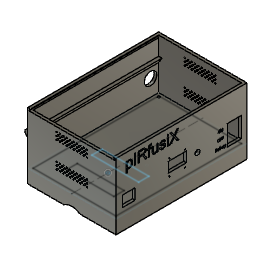
Gateway Enclosure Final Version (Autodesk Fusion 360 design; units mm, degrees)
Autodesk Fusion 360 part; units mm, degrees
(part 1 of 2)
box "BoxPrimitive1" add length 193 width 130 height 77.5 placed x (0, 1, 0) y (-1, 0, 0) z (0, 0, 1) at (80, 0, 0) makes body 1 in component "Box"
shell "Shell1" thickness 4 removed faces 1 at (36.6667, 64.3333, 77.5) on bodies 1 in component "Box"
sketch "Sketch2" plane through (0, 0, 0) normal (0, -1, 0) x (1, 0, 0) in component "Box"
  line L0 (-50, 77.5) -> (-50, 0)
  line L1 (-50, 0) -> (80, 0)
  line L2 (80, 0) -> (80, 77.5)
  line L3 (80, 77.5) -> (-50, 77.5)
  line L4 (76, 77.5) -> (78.2943, 74.2234)
  line L5 (76, 77.5) -> (80, 77.5) construction
  line L6 (15, 77.5) -> (15, 74.2234) construction
  line L7 (15, 74.2234) -> (78.2943, 74.2234)
  line L8 (15, 74.2234) -> (-48.2943, 74.2234)
  line L9 (-46, 77.5) -> (-48.2943, 74.2234)
  point P0 (-46, 77.5)
  point P1 (76, 77.5)
  dimension "d7" = 55
  dimension "d8" = 4
  constraint horizontal L5
  constraint coincident P1 L4.start
  constraint coincident L2.end L3.start
  constraint midpoint L3 L6.start
  constraint perpendicular L3 L6
  constraint horizontal L4.end L6.end
  constraint symmetric P1 L6 P0
  constraint symmetric L4.end L6 L8.end
  constraint symmetric L7.start L6 L8.start
  measures "d7" angle of L4 L5
  measures "d8" distance of P1 L4.end
extrude "Extrude1" cut sketch "Sketch2" against normal up to surface (189 mm away) contours L3 L4 L7 L8 L9 bodies 1 in component "Box"
sketch "Sketch1" plane through (0, 0, 0) normal (0, -1, 0) x (1, 0, 0) in component "Lid"
  line L0 (-48.2943, 74.2234) -> (-46, 77.5)
  line L1 (-46, 77.5) -> (-50, 77.5)
  line L2 (-50, 77.5) -> (-50, 0)
  line L3 (-50, 0) -> (80, 0)
  line L4 (80, 0) -> (80, 77.5)
  line L5 (80, 77.5) -> (76, 77.5)
  line L6 (76, 77.5) -> (78.2943, 74.2234)
  line L7 (78.2943, 74.2234) -> (-48.2943, 74.2234)
  line L8 (-48.2943, 74.2234) -> (-46, 77.5)
  line L9 (78.2943, 74.2234) -> (-48.2943, 74.2234)
  line L10 (-46, 77.5) -> (76, 77.5)
  line L11 (76, 77.5) -> (78.2943, 74.2234)
  line L12 (80, 77.8) -> (75.4237, 77.8)
  line L13 (75.4237, 77.8) -> (77.718, 74.5234)
  line L14 (77.718, 74.5234) -> (-47.718, 74.5234)
  line L15 (-47.718, 74.5234) -> (-45.4237, 77.8)
  line L16 (-45.4237, 77.8) -> (-50, 77.8)
  line L17 (-45.6338, 77.5) -> (75.6338, 77.5)
  dimension "d11" = 0.3
  constraint coincident L10 L17.start
  constraint coincident L15 L17.start
  constraint coincident L13 L17.end
  constraint coincident L10 L17.end
extrude "Extrude1'" add sketch "Sketch1" against normal up to surface (188.7 mm away) separate body contours L10 L13 L14 L15 L17 makes body 2 in component "Lid"
sketch "Sketch2 (2)" plane through (0, 0, 0) normal (0, -1, 0) x (1, 0, 0) in component "Lid"
  line L0 (-45.6338, 77.5) -> (-47.718, 74.5234)
  line L1 (-47.718, 74.5234) -> (77.718, 74.5234)
  line L2 (77.718, 74.5234) -> (75.6338, 77.5)
  line L3 (75.6338, 77.5) -> (-45.6338, 77.5)
  ellipse E0 centre (15, 77.5) end of major axis (22, 77.5) minor radius 0.6667
  line L4 (8, 77.5) -> (22, 77.5)
  line L5 (15, 76.8333) -> (15, 78.1667)
  dimension "d19" = 1.3333
  constraint midpoint L3 E0.centre
  constraint parallel L3 L4
  constraint coincident E0 L4.start
  constraint coincident E0 L4.end
  constraint coincident E0 L5.start
  constraint coincident E0 L5.end
extrude "Extrude2" cut sketch "Sketch2 (2)" along normal blind 5 from surface at -10 contours L3 E0 L4 L5 | L3 E0 L4 L5 | L3 E0 L4 L5 | L3 E0 L4 L5 bodies 2 in component "Lid"
sketch "Sketch3" plane through (80, 0, 0) normal (1, 0, 0) x (0, 1, 0) in component "Box"
  line L0 (0, 77.5) -> (0, 0)
  line L1 (0, 0) -> (193, 0)
  line L2 (193, 0) -> (193, 77.5)
  line L3 (193, 77.5) -> (0, 77.5)
  line L4 (164, 40) -> (185, 40)
  line L5 (185, 40) -> (185, 10)
  line L6 (185, 10) -> (164, 10)
  line L7 (164, 10) -> (164, 40)
  circle A0 centre (120, 25) radius 3.65
  line L8 (77, 35.0926) -> (104, 35.0926)
  line L9 (104, 35.0926) -> (104, 20.0926)
  line L10 (104, 20.0926) -> (77, 20.0926)
  line L11 (77, 20.0926) -> (77, 35.0926)
  circle A1 centre (79, 38.0926) radius 1
  circle A2 centre (79, 15.0926) radius 1
  line L12 (90.5, 41) -> (90.5, 10.3458) construction
  circle A3 centre (102, 38.0926) radius 1
  circle A4 centre (102, 15.0926) radius 1
  line L13 (10, 10) -> (28, 10)
  line L14 (28, 10) -> (28, 26)
  line L15 (28, 26) -> (10, 26)
  line L16 (10, 26) -> (10, 10)
  line L17 (15, 45) -> (125, 45) construction
  line L18 (125, 45) -> (125, 70) construction
  line L19 (125, 70) -> (15, 70) construction
  line L20 (15, 70) -> (15, 45) construction
  line L21 (148.023, 12.1625) -> (160.8666, 12.1744) construction
  line L22 (160.8666, 12.1744) -> (160.8436, 37.0119) construction
  line L23 (160.8436, 37.0119) -> (148, 37) construction
  line L24 (148, 37) -> (148.023, 12.1625) construction
  dimension "d29" = 7.3
  dimension "d30" = 27
  dimension "d31" = 15
  dimension "d32" = 2
  dimension "d33" = 2
  dimension "d58" = 18
  dimension "d59" = 16
  dimension "d66" = 21
  dimension "d67" = 30
  dimension "d627" = 15
  dimension "d654" = 3.5
  text T0 "pIRfusiX" font "Arial" height 15 align left top in box 110 x 25 at (15, 45) x (1, 0) y (0, 1) spacing 1 kerned
  text T1 "ON\n\nOFF\n\nBattery" font "Arial" height 3.5 align centre middle in box 12.8436 x 24.8375 at (148.023, 12.1625) x (1, 0.000925) y (-0.000925, 1) spacing 1 kerned
  constraint horizontal L4
  constraint vertical L5
  constraint horizontal L6
  constraint vertical L7
  constraint horizontal L8
  constraint vertical L9
  constraint horizontal L10
  constraint vertical L11
  constraint perpendicular L10 L12
  constraint symmetric A1 L12 A3
  constraint symmetric A2 L12 A4
  constraint horizontal L13
  constraint vertical L14
  constraint horizontal L15
  constraint vertical L16
  measures "d29" diameter of A0
  measures "d30" distance of L8.start L8.end
  measures "d31" distance of L8.start L10.end
  measures "d32" diameter of A1
  measures "d33" diameter of A2
  measures "d58" distance of L13.start L13.end
  measures "d59" distance of L13.start L15.end
  measures "d66" distance of L4.start L4.end
  measures "d67" distance of L4.start L6.end
  measures "d569" diameter of A3.centre
extrude "Extrude17" cut sketch "Sketch3" against normal blind 1 text T1 bodies 1 in component "Box"
extrude "Extrude14" cut sketch "Sketch3" against normal blind 1 text T0 bodies 1 in component "Box"
extrude "Extrude5" cut sketch "Sketch3" against normal up to surface (4 mm away) contours L13 L14 L15 L16 bodies 1 in component "Box"
extrude "Extrude2'" cut sketch "Sketch3" against normal up to surface (4 mm away) contours L4 L5 L6 L7 | A0 | L8 L9 L10 L11 | A1 | A2 | A3 | A4 bodies 1 in component "Box"
sketch "Sketch4" plane through (-50, 0, 0) normal (-1, 0, 0) x (0, -1, 0) in component "Box"
  line L0 (-193, 77.5) -> (-193, 0)
  line L1 (-193, 0) -> (0, 0)
  line L2 (0, 0) -> (0, 77.5)
  line L3 (0, 77.5) -> (-193, 77.5)
  circle A0 centre (-177, 28) radius 9.25
  line L4 (-15, 15) -> (-25, 15)
  line L5 (-25, 15) -> (-25, 45)
  line L6 (-25, 45) -> (-15, 45)
  line L7 (-15, 45) -> (-15, 15)
  line L8 (-125, 45) -> (-115, 45)
  line L9 (-115, 45) -> (-115, 15)
  line L10 (-115, 15) -> (-125, 15)
  line L11 (-125, 15) -> (-125, 45)
  dimension "d40" = 18.5
  dimension "d115" = 10
  dimension "d116" = 30
  constraint horizontal L4
  constraint vertical L5
  constraint horizontal L6
  constraint vertical L7
  constraint horizontal L8
  constraint vertical L9
  constraint horizontal L10
  constraint vertical L11
  measures "d40" diameter of A0
  measures "d115" distance of L4.start L4.end
  measures "d116" distance of L4.start L6.end
extrude "Extrude10" add sketch "Sketch4" along normal blind 20 contours L8 L9 L10 L11 bodies 1 in component "Box"
extrude "Extrude9" add sketch "Sketch4" along normal blind 20 contours L4 L5 L6 L7 bodies 1 in component "Box"
extrude "Extrude3" cut sketch "Sketch4" against normal up to surface (4 mm away) contours A0 bodies 1 in component "Box"
sketch "Sketch5" plane through (0, 0, 4) normal (0, 0, 1) x (-1, 0, 0) in component "Box"
  line L0 (-76, -189) -> (46, -189)
  line L1 (46, -189) -> (46, -4)
  line L2 (46, -4) -> (-76, -4)
  line L3 (-76, -4) -> (-76, -189)
  circle A0 centre (40.46, -183.46) radius 1.75
  circle A1 centre (-38, -148) radius 1.75
  circle A2 centre (40, -41) radius 1.75
  circle A3 centre (-34, -92) radius 1.75
  dimension "d45" = 3.5
  dimension "d48" = 3.5
  dimension "d51" = 3.5
  dimension "d54" = 3.5
  measures "d45" diameter of A0
  measures "d48" diameter of A1
  measures "d51" diameter of A2
  measures "d54" diameter of A3
extrude "Extrude4" cut sketch "Sketch5" against normal up to surface (4 mm away) contours A0 | A1 | A2 | A3 bodies 1 in component "Box"
sketch "Sketch8" plane through (0, 193, 0) normal (0, 1, 0) x (-1, 0, 0) in component "Box"
  line L0 (-80, 77.5) -> (-80, 0)
  line L1 (-80, 0) -> (50, 0)
  line L2 (50, 0) -> (50, 77.5)
  line L3 (50, 77.5) -> (-80, 77.5)
  line L4 (-71, 50.5) -> (-76, 50.5)
  line L5 (-76, 50.5) -> (-76, 42.5)
  line L6 (-76, 42.5) -> (-71, 50.5)
  line L7 (-15, 77.5) -> (-15, 38.8075) construction
  line L8 (46, 42.5) -> (41, 50.5)
  line L9 (41, 50.5) -> (46, 50.5)
  line L10 (46, 50.5) -> (46, 42.5)
  dimension "d93" = 8
  constraint horizontal L4
  constraint vertical L5
  constraint midpoint L3 L7.start
  constraint perpendicular L3 L7
  constraint symmetric L5.end L7 L8.start
  constraint symmetric L4.start L7 L8.end
  constraint symmetric L4.end L7 L9.end
  measures "d93" distance of L5.end L4.end
extrude "Extrude8" add sketch "Sketch8" against normal up to surface (193 mm away) contours L4 L5 L6 | L8 L9 L10 bodies 1 in component "Box"
sketch "Sketch1 (2)" plane through (-46, 0, 0) normal (1, 0, 0) x (0, 1, 0) in component "Level (1)"
  line L0 (4, 50.5) -> (189, 50.5)
  line L1 (189, 50.5) -> (189, 74.2234)
  line L2 (189, 74.2234) -> (4, 74.2234)
  line L3 (4, 74.2234) -> (4, 50.5)
  line L4 (4.3, 74.2234) -> (4.3, 50.8)
  line L5 (4.3, 50.8) -> (188.7, 50.8)
  line L6 (188.7, 50.8) -> (188.7, 74.2234)
  line L7 (4.3, 54.2) -> (188.7, 54.2)
  constraint coincident L4 L7.start
  constraint coincident L6 L7.end
  constraint perpendicular L6 L7
extrude "Extrude1''" add sketch "Sketch1 (2)" along normal up to surface (121.4 mm away) from surface at 0.3 separate body contours L4 L5 L6 L7 makes body 3 in component "Level (1)"
sketch "Sketch2 (3)" plane through (0, 0, 54.2) normal (0, 0, 1) x (-1, 0, 0) in component "Level (1)"
  line L0 (-75.7, -4.3) -> (-75.7, -188.7)
  line L1 (-75.7, -188.7) -> (45.7, -188.7)
  line L2 (45.7, -188.7) -> (45.7, -4.3)
  line L3 (45.7, -4.3) -> (-75.7, -4.3)
  line L4 (15, -10) -> (15, -4.3)
  line L5 (15, -4.3) -> (-45, -4.3)
  line L6 (-45, -4.3) -> (-45, -24.3)
  line L7 (-45, -24.3) -> (15, -24.3)
  line L8 (15, -24.3) -> (15, -4.3)
  line L9 (-15, -4.3) -> (-15, -160) construction
  line L10 (25, -182.5663) -> (30, -182.5663)
  line L11 (30, -182.5663) -> (30, -167.5663)
  line L12 (30, -167.5663) -> (25, -167.5663)
  line L13 (25, -167.5663) -> (25, -182.5663)
  line L14 (25, -65) -> (30, -65)
  line L15 (30, -65) -> (30, -80)
  line L16 (30, -80) -> (25, -80)
  line L17 (25, -80) -> (25, -65)
  line L18 (-55, -182.5663) -> (-60, -182.5663)
  line L19 (-55, -167.5663) -> (-55, -182.5663)
  line L20 (-60, -182.5663) -> (-60, -167.5663)
  line L21 (-60, -167.5663) -> (-55, -167.5663)
  line L22 (-60, -65) -> (-60, -80)
  line L23 (-60, -80) -> (-55, -80)
  line L24 (-55, -80) -> (-55, -65)
  line L25 (-55, -65) -> (-60, -65)
  dimension "d101" = 60
  dimension "d102" = 20
  dimension "d104" = 5
  dimension "d105" = 15
  dimension "d106" = 5
  dimension "d107" = 15
  constraint coincident L3 L4.end
  constraint perpendicular L3 L4
  constraint horizontal L5
  constraint vertical L6
  constraint horizontal L7
  constraint vertical L8
  constraint midpoint L3 L9.start
  constraint perpendicular L5 L9
  constraint horizontal L10
  constraint vertical L11
  constraint horizontal L12
  constraint vertical L13
  constraint horizontal L14
  constraint vertical L15
  constraint horizontal L16
  constraint vertical L17
  constraint symmetric L9 L10.start L18.start
  constraint symmetric L9 L10.end L18.end
  constraint symmetric L9 L11.end L20.end
  constraint symmetric L9 L12.end L19.start
  constraint symmetric L9 L14.start L24.end
  constraint symmetric L9 L14.end L22.start
  constraint symmetric L9 L15.end L22.end
  constraint symmetric L9 L16.end L23.end
  measures "d101" distance of L4.end L5.end
  measures "d102" distance of L4.end L7.end
  measures "d104" distance of L10.start L10.end
  measures "d105" distance of L10.start L12.end
  measures "d106" distance of L14.start L14.end
  measures "d107" distance of L14.start L16.end
extrude "Extrude2''" cut sketch "Sketch2 (3)" against normal up to surface (3.4 mm away) contours L3 L4 L5 L6 L7 L8 | L10 L11 L12 L13 | L14 L15 L16 L17 | L18 L19 L20 L21 | L22 L23 L24 L25 bodies 3 in component "Level (1)"
sketch "Sketch10" plane through (5.1327, 15, -5.831) normal (0, -1, 0) x (1, 0, 0) in component "Box"
  line L0 (-55.1327, 20.831) -> (-55.1327, 50.831)
  line L1 (-55.1327, 50.831) -> (-75.1327, 50.831)
  line L2 (-75.1327, 50.831) -> (-75.1327, 20.831)
  line L3 (-75.1327, 20.831) -> (-55.1327, 20.831)
  spline S0 degree 2 poles (-55.1327, 20.831) (-82.6327, 35.831) (-55.1327, 50.831) knots 0 0 0 4.88083 4.88083 4.88083 weights 1 2.333333 1
  circle A0 centre (-63.1327, 35.831) radius 5
  dimension "d123" = 10
  constraint coincident L0.end L1.start
  constraint coincident L0.start L3.end
  measures "d123" diameter of A0
extrude "Extrude12" cut sketch "Sketch10" against normal up to surface (110 mm away) contours L1 L2 L3 S0 | A0 bodies 1 in component "Box"
sketch "Sketch1 (3)" plane through (0, 193, 0) normal (0, 1, 0) x (-1, 0, 0)
  line L0 (-80, 77.5) -> (-80, 0)
  line L1 (-80, 0) -> (50, 0)
  line L2 (50, 0) -> (50, 77.5)
  line L3 (50, 77.5) -> (-80, 77.5)
  circle A0 centre (-32.5, 19.5135) radius 1
  circle A1 centre (-27.5, 19.5135) radius 1
  circle A2 centre (-27.5, 19.5135) radius 1
  circle A3 centre (-32.5, 19.5135) radius 1
  circle A4 centre (-35, 22.0135) radius 1
  circle A5 centre (-35, 22.0135) radius 1
  circle A6 centre (-35, 22.0135) radius 1
  circle A7 centre (-30, 22.0135) radius 1
  circle A8 centre (-30, 22.0135) radius 1
  circle A9 centre (-35, 22.0135) radius 1
  circle A10 centre (-32.5, 24.5135) radius 1
  circle A11 centre (-35, 27.0135) radius 1
  circle A12 centre (-35, 27.0135) radius 1
  circle A13 centre (-30, 27.0135) radius 1
  circle A14 centre (-35, 22.0135) radius 1
  circle A15 centre (-30, 27.0135) radius 1
  circle A16 centre (-35, 22.0135) radius 1
  circle A17 centre (-32.5, 24.5135) radius 1
  circle A18 centre (-32.5, 19.5135) radius 1
  circle A19 centre (-27.5, 19.5135) radius 1
  circle A20 centre (-27.5, 19.5135) radius 1
  circle A21 centre (-32.5, 19.5135) radius 1
  circle A22 centre (-35, 22.0135) radius 1
  circle A23 centre (-35, 22.0135) radius 1
  circle A24 centre (-30, 22.0135) radius 1
  circle A25 centre (-35, 27.0135) radius 1
  circle A26 centre (-30, 27.0135) radius 1
  circle A27 centre (-35, 22.0135) radius 1
  circle A28 centre (-35, 22.0135) radius 1
  circle A29 centre (-35, 22.0135) radius 1
  circle A30 centre (-35, 22.0135) radius 1
  circle A31 centre (-32.5, 24.5135) radius 1
  circle A32 centre (-35, 27.0135) radius 1
  circle A33 centre (-30, 22.0135) radius 1
  circle A34 centre (-30, 27.0135) radius 1
  circle A35 centre (-32.5, 24.5135) radius 1
  circle A36 centre (-2.5, 24.5135) radius 1
  circle A37 centre (-22.5, 19.5135) radius 1
  circle A38 centre (2.5, 29.5135) radius 1
  circle A39 centre (-7.5, 19.5135) radius 1
  circle A40 centre (2.5, 19.5135) radius 1
  circle A41 centre (-17.5, 19.5135) radius 1
  circle A42 centre (-10, 22.0135) radius 1
  circle A43 centre (-17.5, 19.5135) radius 1
  circle A44 centre (-22.5, 19.5135) radius 1
  circle A45 centre (-25, 22.0135) radius 1
  circle A46 centre (-25, 22.0135) radius 1
  circle A47 centre (-20, 22.0135) radius 1
  circle A48 centre (-25, 27.0135) radius 1
  circle A49 centre (-20, 27.0135) radius 1
  circle A50 centre (2.5, 24.5135) radius 1
  circle A51 centre (-7.5, 24.5135) radius 1
  circle A52 centre (-25, 22.0135) radius 1
  circle A53 centre (-25, 22.0135) radius 1
  circle A54 centre (-25, 22.0135) radius 1
  circle A55 centre (-25, 22.0135) radius 1
  circle A56 centre (-22.5, 24.5135) radius 1
  circle A57 centre (-25, 27.0135) radius 1
  circle A58 centre (-20, 22.0135) radius 1
  circle A59 centre (-20, 27.0135) radius 1
  circle A60 centre (-22.5, 24.5135) radius 1
  circle A61 centre (-27.5, 24.5135) radius 1
  circle A62 centre (7.5, 19.5135) radius 1
  circle A63 centre (-17.5, 24.5135) radius 1
  circle A64 centre (-37.5, 24.5135) radius 1
  circle A65 centre (-37.5, 19.5135) radius 1
  circle A66 centre (-15, 27.0135) radius 1
  circle A67 centre (-32.5, 29.5135) radius 1
  circle A68 centre (-37.5, 29.5135) radius 1
  circle A69 centre (-27.5, 29.5135) radius 1
  circle A70 centre (-22.5, 29.5135) radius 1
  circle A71 centre (-17.5, 29.5135) radius 1
  circle A72 centre (-35, 22.0135) radius 1
  circle A73 centre (-27.5, 29.5135) radius 1
  circle A74 centre (-17.5, 29.5135) radius 1
  circle A75 centre (-20, 22.0135) radius 1
  circle A76 centre (-35, 22.0135) radius 1
  circle A77 centre (-35, 27.0135) radius 1
  circle A78 centre (-35, 22.0135) radius 1
  circle A79 centre (-35, 22.0135) radius 1
  circle A80 centre (-37.5, 24.5135) radius 1
  circle A81 centre (-35, 22.0135) radius 1
  circle A82 centre (-35, 22.0135) radius 1
  circle A83 centre (-25, 22.0135) radius 1
  circle A84 centre (-20, 27.0135) radius 1
  circle A85 centre (-35, 22.0135) radius 1
  circle A86 centre (-32.5, 24.5135) radius 1
  circle A87 centre (-37.5, 29.5135) radius 1
  circle A88 centre (-35, 27.0135) radius 1
  circle A89 centre (-35, 22.0135) radius 1
  circle A90 centre (-27.5, 24.5135) radius 1
  circle A91 centre (-35, 22.0135) radius 1
  circle A92 centre (-35, 27.0135) radius 1
  circle A93 centre (-20, 27.0135) radius 1
  circle A94 centre (-35, 22.0135) radius 1
  circle A95 centre (-35, 27.0135) radius 1
  circle A96 centre (-35, 22.0135) radius 1
  circle A97 centre (-35, 22.0135) radius 1
  circle A98 centre (-22.5, 24.5135) radius 1
  circle A99 centre (-25, 22.0135) radius 1
  circle A100 centre (-25, 27.0135) radius 1
  circle A101 centre (-32.5, 24.5135) radius 1
  circle A102 centre (-32.5, 19.5135) radius 1
  circle A103 centre (-30, 22.0135) radius 1
  circle A104 centre (-25, 27.0135) radius 1
  circle A105 centre (-30, 22.0135) radius 1
  circle A106 centre (-25, 22.0135) radius 1
  circle A107 centre (-20, 22.0135) radius 1
  circle A108 centre (-25, 22.0135) radius 1
  circle A109 centre (-30, 22.0135) radius 1
  circle A110 centre (-17.5, 24.5135) radius 1
  circle A111 centre (-30, 27.0135) radius 1
  circle A112 centre (-32.5, 24.5135) radius 1
  circle A113 centre (-30, 27.0135) radius 1
  circle A114 centre (-30, 27.0135) radius 1
  circle A115 centre (-25, 22.0135) radius 1
  circle A116 centre (-30, 27.0135) radius 1
  circle A117 centre (-32.5, 24.5135) radius 1
  circle A118 centre (-30, 22.0135) radius 1
  circle A119 centre (-22.5, 24.5135) radius 1
  circle A120 centre (-32.5, 29.5135) radius 1
  circle A121 centre (-22.5, 29.5135) radius 1
  circle A122 centre (-25, 22.0135) radius 1
  circle A123 centre (-2.5, 29.5135) radius 1
  circle A124 centre (-2.5, 19.5135) radius 1
  circle A125 centre (-17.5, 19.5135) radius 1
  circle A126 centre (5, 27.0135) radius 1
  circle A127 centre (-22.5, 19.5135) radius 1
  circle A128 centre (0, 22.0135) radius 1
  circle A129 centre (-22.5, 19.5135) radius 1
  circle A130 centre (7.5, 29.5135) radius 1
  circle A131 centre (5, 22.0135) radius 1
  circle A132 centre (7.5, 24.5135) radius 1
  circle A133 centre (-27.5, 19.5135) radius 1
  circle A134 centre (-27.5, 19.5135) radius 1
  circle A135 centre (0, 27.0135) radius 1
  circle A136 centre (-17.5, 19.5135) radius 1
  circle A137 centre (-27.5, 19.5135) radius 1
  circle A138 centre (-12.5, 24.5135) radius 1
  circle A139 centre (-32.5, 19.5135) radius 1
  circle A140 centre (-15, 22.0135) radius 1
  circle A141 centre (-27.5, 19.5135) radius 1
  circle A142 centre (-32.5, 19.5135) radius 1
  circle A143 centre (-7.5, 29.5135) radius 1
  circle A144 centre (-32.5, 19.5135) radius 1
  circle A145 centre (-37.5, 19.5135) radius 1
  circle A146 centre (-12.5, 19.5135) radius 1
  circle A147 centre (-5, 22.0135) radius 1
  circle A148 centre (-12.5, 29.5135) radius 1
  circle A149 centre (-10, 27.0135) radius 1
  circle A150 centre (-5, 27.0135) radius 1
  circle A151 centre (-25, 22.0135) radius 1
  circle A152 centre (-30, 22.0135) radius 1
  circle A153 centre (-25, 22.0135) radius 1
  circle A154 centre (-25, 22.0135) radius 1
  circle A155 centre (-27.5, 19.5135) radius 1
  circle A156 centre (-25, 22.0135) radius 1
  circle A157 centre (-27.5, 19.5135) radius 1
  circle A158 centre (-27.5, 19.5135) radius 1
  circle A159 centre (-27.5, 19.5135) radius 1
  circle A160 centre (-25, 22.0135) radius 1
  circle A161 centre (-25, 22.0135) radius 1
  circle A162 centre (-25, 22.0135) radius 1
  circle A163 centre (-27.5, 19.5135) radius 1
  circle A164 centre (-7.5, 19.5135) radius 1
  circle A165 centre (-27.5, 19.5135) radius 1
  circle A166 centre (-25, 22.0135) radius 1
  circle A167 centre (-25, 22.0135) radius 1
  circle A168 centre (-25, 22.0135) radius 1
  circle A169 centre (-25, 22.0135) radius 1
  circle A170 centre (-27.5, 19.5135) radius 1
  circle A171 centre (-25, 22.0135) radius 1
  circle A172 centre (-27.5, 19.5135) radius 1
  circle A173 centre (-32.5, 19.5135) radius 1
  circle A174 centre (-30, 22.0135) radius 1
  circle A175 centre (-32.5, 19.5135) radius 1
  circle A176 centre (-17.5, 19.5135) radius 1
  circle A177 centre (5, 22.0135) radius 1
  circle A178 centre (-22.5, 19.5135) radius 1
  circle A179 centre (-22.5, 19.5135) radius 1
  circle A180 centre (2.5, 19.5135) radius 1
  circle A181 centre (-20, 22.0135) radius 1
  circle A182 centre (-10, 22.0135) radius 1
  circle A183 centre (-20, 22.0135) radius 1
  circle A184 centre (-20, 22.0135) radius 1
  circle A185 centre (-2.5, 19.5135) radius 1
  circle A186 centre (-5, 22.0135) radius 1
  circle A187 centre (-22.5, 19.5135) radius 1
  circle A188 centre (0, 22.0135) radius 1
  circle A189 centre (7.5, 19.5135) radius 1
  circle A190 centre (-20, 22.0135) radius 1
  circle A191 centre (-12.5, 19.5135) radius 1
  circle A192 centre (-17.5, 19.5135) radius 1
  circle A193 centre (-22.5, 19.5135) radius 1
  circle A194 centre (-17.5, 19.5135) radius 1
  circle A195 centre (-17.5, 19.5135) radius 1
  circle A196 centre (-15, 22.0135) radius 1
  circle A197 centre (-35, 22.0135) radius 1
  circle A198 centre (-35, 22.0135) radius 1
  circle A199 centre (-32.5, 19.5135) radius 1
  circle A200 centre (-30, 22.0135) radius 1
  circle A201 centre (-35, 22.0135) radius 1
  circle A202 centre (-35, 22.0135) radius 1
  circle A203 centre (-35, 22.0135) radius 1
  circle A204 centre (-30, 22.0135) radius 1
  circle A205 centre (-32.5, 19.5135) radius 1
  circle A206 centre (-35, 22.0135) radius 1
  circle A207 centre (-32.5, 19.5135) radius 1
  circle A208 centre (-30, 22.0135) radius 1
  circle A209 centre (-32.5, 19.5135) radius 1
  circle A210 centre (-32.5, 19.5135) radius 1
  circle A211 centre (-35, 22.0135) radius 1
  circle A212 centre (-35, 22.0135) radius 1
  circle A213 centre (-30, 22.0135) radius 1
  circle A214 centre (-35, 22.0135) radius 1
  circle A215 centre (-35, 22.0135) radius 1
  circle A216 centre (-37.5, 19.5135) radius 1
  circle A217 centre (-30, 22.0135) radius 1
  circle A218 centre (-35, 22.0135) radius 1
  circle A219 centre (-35, 22.0135) radius 1
  circle A220 centre (-35, 22.0135) radius 1
  circle A221 centre (-32.5, 19.5135) radius 1
  circle A222 centre (-35, 22.0135) radius 1
  circle A223 centre (-30, 22.0135) radius 1
  circle A224 centre (-35, 22.0135) radius 1
  circle A225 centre (-35, 22.0135) radius 1
  circle A226 centre (-35, 22.0135) radius 1
  circle A227 centre (-35, 22.0135) radius 1
  circle A228 centre (-7.5, 29.5135) radius 1
  circle A229 centre (-20, 27.0135) radius 1
  circle A230 centre (-22.5, 29.5135) radius 1
  circle A231 centre (-35, 22.0135) radius 1
  circle A232 centre (-35, 22.0135) radius 1
  circle A233 centre (-35, 22.0135) radius 1
  circle A234 centre (-15, 27.0135) radius 1
  circle A235 centre (-35, 22.0135) radius 1
  circle A236 centre (-5, 27.0135) radius 1
  circle A237 centre (-20, 27.0135) radius 1
  circle A238 centre (-2.5, 29.5135) radius 1
  circle A239 centre (-37.5, 19.5135) radius 1
  circle A240 centre (-35, 22.0135) radius 1
  circle A241 centre (-35, 22.0135) radius 1
  circle A242 centre (-10, 27.0135) radius 1
  circle A243 centre (5, 27.0135) radius 1
  circle A244 centre (-27.5, 24.5135) radius 1
  circle A245 centre (-22.5, 24.5135) radius 1
  circle A246 centre (-17.5, 29.5135) radius 1
  circle A247 centre (-27.5, 29.5135) radius 1
  circle A248 centre (-37.5, 24.5135) radius 1
  circle A249 centre (-35, 27.0135) radius 1
  circle A250 centre (-22.5, 24.5135) radius 1
  circle A251 centre (-12.5, 24.5135) radius 1
  circle A252 centre (-35, 27.0135) radius 1
  circle A253 centre (-30, 27.0135) radius 1
  circle A254 centre (-32.5, 24.5135) radius 1
  circle A255 centre (-32.5, 24.5135) radius 1
  circle A256 centre (-20, 27.0135) radius 1
  circle A257 centre (-25, 27.0135) radius 1
  circle A258 centre (-30, 27.0135) radius 1
  circle A259 centre (-25, 27.0135) radius 1
  circle A260 centre (-12.5, 29.5135) radius 1
  circle A261 centre (-35, 27.0135) radius 1
  circle A262 centre (-30, 27.0135) radius 1
  circle A263 centre (-35, 27.0135) radius 1
  circle A264 centre (-35, 27.0135) radius 1
  circle A265 centre (-35, 27.0135) radius 1
  circle A266 centre (-30, 27.0135) radius 1
  circle A267 centre (-30, 27.0135) radius 1
  circle A268 centre (-22.5, 24.5135) radius 1
  circle A269 centre (-32.5, 24.5135) radius 1
  circle A270 centre (-35, 27.0135) radius 1
  circle A271 centre (-37.5, 29.5135) radius 1
  circle A272 centre (-7.5, 24.5135) radius 1
  circle A273 centre (-32.5, 29.5135) radius 1
  circle A274 centre (-20, 27.0135) radius 1
  circle A275 centre (7.5, 24.5135) radius 1
  circle A276 centre (-25, 27.0135) radius 1
  circle A277 centre (2.5, 29.5135) radius 1
  circle A278 centre (-27.5, 29.5135) radius 1
  circle A279 centre (-30, 27.0135) radius 1
  circle A280 centre (-35, 27.0135) radius 1
  circle A281 centre (-17.5, 29.5135) radius 1
  circle A282 centre (-37.5, 24.5135) radius 1
  circle A283 centre (-32.5, 24.5135) radius 1
  circle A284 centre (-27.5, 24.5135) radius 1
  circle A285 centre (-30, 27.0135) radius 1
  circle A286 centre (0, 27.0135) radius 1
  circle A287 centre (-32.5, 29.5135) radius 1
  circle A288 centre (7.5, 29.5135) radius 1
  circle A289 centre (-22.5, 29.5135) radius 1
  circle A290 centre (-25, 27.0135) radius 1
  circle A291 centre (-30, 27.0135) radius 1
  circle A292 centre (-37.5, 29.5135) radius 1
  circle A293 centre (-17.5, 24.5135) radius 1
  circle A294 centre (-17.5, 24.5135) radius 1
  circle A295 centre (2.5, 24.5135) radius 1
  circle A296 centre (-2.5, 24.5135) radius 1
  circle A297 centre (-32.5, 24.5135) radius 1
  circle A298 centre (-32.5, 24.5135) radius 1
  circle A299 centre (-22.5, 24.5135) radius 1
  circle A300 centre (-32.5, 24.5135) radius 1
  circle A301 centre (-32.5, 24.5135) radius 1
  circle A302 centre (-25, 60) radius 1
  circle A303 centre (-30, 60) radius 1
  circle A304 centre (-25, 60) radius 1
  circle A305 centre (-25, 60) radius 1
  circle A306 centre (-27.5, 57.5) radius 1
  circle A307 centre (-25, 60) radius 1
  circle A308 centre (-27.5, 57.5) radius 1
  circle A309 centre (-27.5, 57.5) radius 1
  circle A310 centre (-27.5, 57.5) radius 1
  circle A311 centre (-25, 60) radius 1
  circle A312 centre (-25, 60) radius 1
  circle A313 centre (-25, 60) radius 1
  circle A314 centre (-27.5, 57.5) radius 1
  circle A315 centre (-7.5, 57.5) radius 1
  circle A316 centre (-27.5, 57.5) radius 1
  circle A317 centre (-25, 60) radius 1
  circle A318 centre (-25, 60) radius 1
  circle A319 centre (-25, 60) radius 1
  circle A320 centre (-25, 60) radius 1
  circle A321 centre (-27.5, 57.5) radius 1
  circle A322 centre (-25, 60) radius 1
  circle A323 centre (-27.5, 57.5) radius 1
  circle A324 centre (-32.5, 57.5) radius 1
  circle A325 centre (-30, 60) radius 1
  circle A326 centre (-32.5, 57.5) radius 1
  circle A327 centre (-17.5, 57.5) radius 1
  circle A328 centre (5, 60) radius 1
  circle A329 centre (-22.5, 57.5) radius 1
  circle A330 centre (-22.5, 57.5) radius 1
  circle A331 centre (2.5, 57.5) radius 1
  circle A332 centre (-20, 60) radius 1
  circle A333 centre (-10, 60) radius 1
  circle A334 centre (-20, 60) radius 1
  circle A335 centre (-20, 60) radius 1
  circle A336 centre (-2.5, 57.5) radius 1
  circle A337 centre (-5, 60) radius 1
  circle A338 centre (-22.5, 57.5) radius 1
  circle A339 centre (0, 60) radius 1
  circle A340 centre (7.5, 57.5) radius 1
  circle A341 centre (-20, 60) radius 1
  circle A342 centre (-12.5, 57.5) radius 1
  circle A343 centre (-17.5, 57.5) radius 1
  circle A344 centre (-22.5, 57.5) radius 1
  circle A345 centre (-17.5, 57.5) radius 1
  circle A346 centre (-17.5, 57.5) radius 1
  circle A347 centre (-15, 60) radius 1
  circle A348 centre (-35, 60) radius 1
  circle A349 centre (-35, 60) radius 1
  circle A350 centre (-32.5, 57.5) radius 1
  circle A351 centre (-30, 60) radius 1
  circle A352 centre (-35, 60) radius 1
  circle A353 centre (-35, 60) radius 1
  circle A354 centre (-35, 60) radius 1
  circle A355 centre (-30, 60) radius 1
  circle A356 centre (-32.5, 57.5) radius 1
  circle A357 centre (-35, 60) radius 1
  circle A358 centre (-32.5, 57.5) radius 1
  circle A359 centre (-30, 60) radius 1
  circle A360 centre (-32.5, 57.5) radius 1
  circle A361 centre (-32.5, 57.5) radius 1
  circle A362 centre (-35, 60) radius 1
  circle A363 centre (-35, 60) radius 1
  circle A364 centre (-30, 60) radius 1
  circle A365 centre (-35, 60) radius 1
  circle A366 centre (-35, 60) radius 1
  circle A367 centre (-37.5, 57.5) radius 1
  circle A368 centre (-30, 60) radius 1
  circle A369 centre (-35, 60) radius 1
  circle A370 centre (-35, 60) radius 1
  circle A371 centre (-35, 60) radius 1
  circle A372 centre (-32.5, 57.5) radius 1
  circle A373 centre (-35, 60) radius 1
  circle A374 centre (-30, 60) radius 1
  circle A375 centre (-35, 60) radius 1
  circle A376 centre (-35, 60) radius 1
  circle A377 centre (-35, 60) radius 1
  circle A378 centre (-35, 60) radius 1
  circle A379 centre (-7.5, 67.5) radius 1
  circle A380 centre (-20, 65) radius 1
  circle A381 centre (-22.5, 67.5) radius 1
  circle A382 centre (-35, 60) radius 1
  circle A383 centre (-35, 60) radius 1
  circle A384 centre (-35, 60) radius 1
  circle A385 centre (-15, 65) radius 1
  circle A386 centre (-35, 60) radius 1
  circle A387 centre (-5, 65) radius 1
  circle A388 centre (-20, 65) radius 1
  circle A389 centre (-2.5, 67.5) radius 1
  circle A390 centre (-37.5, 57.5) radius 1
  circle A391 centre (-35, 60) radius 1
  circle A392 centre (-35, 60) radius 1
  circle A393 centre (-10, 65) radius 1
  circle A394 centre (5, 65) radius 1
  circle A395 centre (-27.5, 62.5) radius 1
  circle A396 centre (-22.5, 62.5) radius 1
  circle A397 centre (-17.5, 67.5) radius 1
  circle A398 centre (-27.5, 67.5) radius 1
  circle A399 centre (-37.5, 62.5) radius 1
  circle A400 centre (-35, 65) radius 1
  circle A401 centre (-22.5, 62.5) radius 1
  circle A402 centre (-12.5, 62.5) radius 1
  circle A403 centre (-35, 65) radius 1
  circle A404 centre (-30, 65) radius 1
  circle A405 centre (-32.5, 62.5) radius 1
  circle A406 centre (-32.5, 62.5) radius 1
  circle A407 centre (-20, 65) radius 1
  circle A408 centre (-25, 65) radius 1
  circle A409 centre (-30, 65) radius 1
  circle A410 centre (-25, 65) radius 1
  circle A411 centre (-12.5, 67.5) radius 1
  circle A412 centre (-35, 65) radius 1
  circle A413 centre (-30, 65) radius 1
  circle A414 centre (-35, 65) radius 1
  circle A415 centre (-35, 65) radius 1
  circle A416 centre (-35, 65) radius 1
  circle A417 centre (-30, 65) radius 1
  circle A418 centre (-30, 65) radius 1
  circle A419 centre (-22.5, 62.5) radius 1
  circle A420 centre (-32.5, 62.5) radius 1
  circle A421 centre (-35, 65) radius 1
  circle A422 centre (-37.5, 67.5) radius 1
  circle A423 centre (-7.5, 62.5) radius 1
  circle A424 centre (-32.5, 67.5) radius 1
  circle A425 centre (-20, 65) radius 1
  circle A426 centre (7.5, 62.5) radius 1
  circle A427 centre (-25, 65) radius 1
  circle A428 centre (2.5, 67.5) radius 1
  circle A429 centre (-27.5, 67.5) radius 1
  circle A430 centre (-30, 65) radius 1
  circle A431 centre (-35, 65) radius 1
  circle A432 centre (-17.5, 67.5) radius 1
  circle A433 centre (-37.5, 62.5) radius 1
  circle A434 centre (-32.5, 62.5) radius 1
  circle A435 centre (-27.5, 62.5) radius 1
  circle A436 centre (-30, 65) radius 1
  circle A437 centre (0, 65) radius 1
  circle A438 centre (-32.5, 67.5) radius 1
  circle A439 centre (7.5, 67.5) radius 1
  circle A440 centre (-22.5, 67.5) radius 1
  circle A441 centre (-25, 65) radius 1
  circle A442 centre (-30, 65) radius 1
  circle A443 centre (-37.5, 67.5) radius 1
  circle A444 centre (-17.5, 62.5) radius 1
  circle A445 centre (-17.5, 62.5) radius 1
  circle A446 centre (2.5, 62.5) radius 1
  circle A447 centre (-2.5, 62.5) radius 1
  circle A448 centre (-32.5, 62.5) radius 1
  circle A449 centre (-32.5, 62.5) radius 1
  circle A450 centre (-22.5, 62.5) radius 1
  circle A451 centre (-32.5, 62.5) radius 1
  circle A452 centre (-32.5, 62.5) radius 1
  dimension "d131" = 2
  dimension "d132" = 2
  dimension "d138" = 2
  dimension "d139" = 2
  dimension "d142" = 2
  dimension "d143" = 2
  dimension "d144" = 2
  dimension "d145" = 2
  dimension "d146" = 2
  dimension "d147" = 2
  dimension "d148" = 2
  dimension "d149" = 2
  dimension "d150" = 2
  dimension "d151" = 2
  dimension "d152" = 2
  dimension "d153" = 2
  dimension "d154" = 2
  dimension "d155" = 2
  dimension "d159" = 2
  dimension "d160" = 2
  dimension "d166" = 2
  dimension "d167" = 2
  dimension "d170" = 2
  dimension "d171" = 2
  dimension "d172" = 2
  dimension "d173" = 2
  dimension "d174" = 2
  dimension "d175" = 2
  dimension "d176" = 2
  dimension "d177" = 2
  dimension "d178" = 2
  dimension "d179" = 2
  dimension "d180" = 2
  dimension "d181" = 2
  dimension "d182" = 2
  dimension "d183" = 2
  dimension "d185" = 2
  dimension "d187" = 2
  dimension "d188" = 2
  dimension "d189" = 2
  dimension "d190" = 2
  dimension "d191" = 2
  dimension "d192" = 2
  dimension "d194" = 2
  dimension "d195" = 2
  dimension "d196" = 2
  dimension "d197" = 2
  dimension "d198" = 2
  dimension "d199" = 2
  dimension "d200" = 2
  dimension "d201" = 2
  dimension "d202" = 2
  dimension "d203" = 2
  dimension "d204" = 2
  dimension "d205" = 2
  dimension "d206" = 2
  dimension "d207" = 2
  dimension "d208" = 2
  dimension "d209" = 2
  dimension "d210" = 2
  dimension "d211" = 2
  dimension "d212" = 2
  dimension "d213" = 2
  dimension "d215" = 2
  dimension "d216" = 2
  dimension "d217" = 2
  dimension "d218" = 2
  dimension "d219" = 2
  dimension "d220" = 2
  dimension "d221" = 2
  dimension "d222" = 2
  dimension "d223" = 2
  dimension "d224" = 2
  dimension "d225" = 2
  dimension "d226" = 2
  dimension "d227" = 2
  dimension "d228" = 2
  dimension "d231" = 2
  dimension "d233" = 2
  dimension "d234" = 2
  dimension "d235" = 2
  dimension "d238" = 2
  dimension "d239" = 2
  dimension "d240" = 2
  dimension "d241" = 2
  dimension "d242" = 2
  dimension "d243" = 2
  dimension "d244" = 2
  dimension "d245" = 2
  dimension "d246" = 2
  dimension "d247" = 2
  dimension "d248" = 2
  dimension "d249" = 2
  dimension "d250" = 2
  dimension "d251" = 2
  dimension "d252" = 2
  dimension "d253" = 2
  dimension "d254" = 2
  dimension "d255" = 2
  dimension "d256" = 2
  dimension "d261" = 2
  dimension "d262" = 2
  dimension "d263" = 2
  dimension "d265" = 2
  dimension "d266" = 2
  dimension "d267" = 2
  dimension "d268" = 2
  dimension "d269" = 2
  dimension "d270" = 2
  dimension "d271" = 2
  dimension "d272" = 2
  dimension "d273" = 2
  dimension "d274" = 2
  dimension "d275" = 2
  dimension "d276" = 2
  dimension "d277" = 2
  dimension "d278" = 2
  dimension "d279" = 2
  dimension "d283" = 2
  dimension "d284" = 2
  dimension "d285" = 2
  dimension "d286" = 2
  dimension "d290" = 2
  dimension "d291" = 2
  dimension "d292" = 2
  dimension "d293" = 2
  dimension "d294" = 2
  dimension "d295" = 2
  dimension "d296" = 2
  dimension "d297" = 2
  dimension "d298" = 2
  dimension "d299" = 2
  dimension "d300" = 2
  dimension "d301" = 2
  dimension "d302" = 2
  dimension "d303" = 2
  dimension "d304" = 2
  dimension "d305" = 2
  dimension "d306" = 2
  dimension "d307" = 2
  dimension "d308" = 2
  dimension "d309" = 2
  dimension "d311" = 2
  dimension "d312" = 2
  dimension "d313" = 2
  dimension "d314" = 2
  dimension "d315" = 2
  dimension "d316" = 2
  dimension "d317" = 2
  dimension "d318" = 2
  dimension "d319" = 2
  dimension "d320" = 5
  dimension "d321" = 2
  dimension "d322" = 2
  dimension "d323" = 2
  dimension "d324" = 2
  dimension "d325" = 2
  dimension "d326" = 2
  dimension "d327" = 2
  dimension "d328" = 2
  dimension "d329" = 2
  dimension "d330" = 2
  dimension "d331" = 2
  dimension "d332" = 2
  dimension "d333" = 2
  dimension "d334" = 2
  dimension "d335" = 2
  dimension "d336" = 2
  dimension "d337" = 2
  dimension "d338" = 2
  dimension "d339" = 2
  dimension "d340" = 2
  dimension "d341" = 2
  dimension "d342" = 2
  dimension "d343" = 2
  dimension "d344" = 2
  dimension "d345" = 2
  dimension "d346" = 2
  dimension "d347" = 2
  dimension "d348" = 2
  dimension "d349" = 2
  dimension "d350" = 2
  dimension "d351" = 2
  dimension "d352" = 2
  dimension "d353" = 2
  dimension "d354" = 2
  dimension "d355" = 2
  dimension "d356" = 2
  dimension "d357" = 2
  dimension "d358" = 2
  dimension "d359" = 2
  dimension "d360" = 2
  dimension "d361" = 2
  dimension "d362" = 2
  dimension "d363" = 2
  dimension "d364" = 2
  dimension "d365" = 2
  dimension "d366" = 2
  dimension "d367" = 2
  dimension "d368" = 2
  dimension "d369" = 2
  dimension "d370" = 2
  dimension "d371" = 2
  dimension "d372" = 2
  dimension "d373" = 2
  dimension "d374" = 2
  dimension "d375" = 2
  dimension "d376" = 2
  dimension "d377" = 2
  dimension "d378" = 2
  dimension "d379" = 2
  dimension "d380" = 2
  dimension "d381" = 2
  dimension "d382" = 2
  dimension "d383" = 2
  dimension "d384" = 2
  dimension "d385" = 2
  dimension "d386" = 2
  dimension "d387" = 2
  dimension "d388" = 2
  dimension "d389" = 2
  dimension "d390" = 2
  dimension "d391" = 2
  dimension "d392" = 2
  dimension "d393" = 2
  dimension "d394" = 2
  dimension "d395" = 2
  dimension "d396" = 2
  dimension "d397" = 2
  dimension "d398" = 2
  dimension "d399" = 2
  dimension "d400" = 2
  dimension "d401" = 2
  dimension "d402" = 2
  dimension "d403" = 2
  dimension "d404" = 2
  dimension "d405" = 2
  dimension "d406" = 2
  dimension "d407" = 2
  dimension "d408" = 2
  dimension "d409" = 2
  dimension "d410" = 2
  dimension "d411" = 2
  dimension "d412" = 2
  dimension "d413" = 2
  dimension "d414" = 2
  dimension "d415" = 2
  dimension "d416" = 2
  dimension "d417" = 2
  dimension "d418" = 2
  dimension "d419" = 2
  dimension "d420" = 2
  dimension "d421" = 2
  dimension "d422" = 2
  dimension "d423" = 2
  dimension "d424" = 2
  dimension "d425" = 2
  dimension "d426" = 2
  dimension "d427" = 2
  dimension "d428" = 2
  dimension "d429" = 2
  dimension "d430" = 2
  dimension "d431" = 2
  dimension "d432" = 2
  dimension "d433" = 2
  dimension "d434" = 2
  dimension "d435" = 2
  dimension "d436" = 2
  dimension "d437" = 2
  dimension "d438" = 2
  dimension "d439" = 2
  dimension "d440" = 2
  dimension "d441" = 2
  dimension "d442" = 2
  dimension "d443" = 2
  dimension "d444" = 2
  dimension "d445" = 2
  dimension "d446" = 2
  dimension "d447" = 2
  dimension "d448" = 2
  dimension "d449" = 2
  dimension "d450" = 2
  dimension "d451" = 2
  dimension "d452" = 2
  dimension "d453" = 2
  dimension "d454" = 2
  dimension "d455" = 2
  dimension "d456" = 2
  dimension "d457" = 2
  dimension "d458" = 2
  dimension "d459" = 2
  dimension "d460" = 2
  dimension "d461" = 2
  dimension "d462" = 2
  dimension "d463" = 2
  dimension "d464" = 2
  dimension "d465" = 2
  dimension "d466" = 2
  dimension "d467" = 2
  dimension "d468" = 2
  dimension "d469" = 2
  dimension "d470" = 2
  dimension "d471" = 2
  dimension "d472" = 5
  dimension "d473" = 2
  dimension "d474" = 2
  dimension "d475" = 2
  dimension "d476" = 2
  dimension "d477" = 2
  dimension "d478" = 2
  dimension "d479" = 2
  dimension "d480" = 2
  dimension "d481" = 2
  dimension "d482" = 2
  dimension "d483" = 2
  dimension "d484" = 2
  dimension "d485" = 2
  dimension "d486" = 2
  dimension "d487" = 2
  dimension "d488" = 2
  dimension "d489" = 2
  dimension "d490" = 2
  dimension "d491" = 2
  dimension "d492" = 2
  dimension "d493" = 2
  dimension "d494" = 2
  dimension "d495" = 2
  dimension "d496" = 2
  dimension "d497" = 2
  dimension "d498" = 2
  dimension "d499" = 2
  dimension "d500" = 2
  dimension "d501" = 2
  dimension "d502" = 2
  dimension "d503" = 2
  dimension "d504" = 2
  dimension "d505" = 2
  dimension "d506" = 2
  dimension "d507" = 2
  dimension "d508" = 2
  dimension "d509" = 2
  dimension "d510" = 2
  dimension "d511" = 2
  dimension "d512" = 2
  dimension "d513" = 2
  dimension "d514" = 2
  dimension "d515" = 2
  dimension "d516" = 2
  dimension "d517" = 2
  dimension "d518" = 2
  dimension "d519" = 2
  dimension "d520" = 2
  dimension "d521" = 2
  dimension "d522" = 2
  dimension "d523" = 2
  dimension "d524" = 2
  dimension "d525" = 2
  dimension "d526" = 2
  dimension "d527" = 2
  dimension "d528" = 2
  dimension "d529" = 2
  dimension "d530" = 2
  dimension "d531" = 2
  dimension "d532" = 2
  dimension "d533" = 2
  dimension "d534" = 2
  dimension "d535" = 2
  dimension "d536" = 2
  dimension "d537" = 2
  dimension "d538" = 2
  dimension "d539" = 2
  dimension "d540" = 2
  dimension "d541" = 2
  dimension "d542" = 2
  dimension "d543" = 2
  dimension "d544" = 2
  dimension "d545" = 2
  dimension "d546" = 2
  dimension "d547" = 2
  dimension "d548" = 2
  dimension "d549" = 2
  dimension "d550" = 2
  dimension "d551" = 2
  dimension "d552" = 2
  dimension "d553" = 2
  dimension "d554" = 2
  dimension "d555" = 2
  dimension "d556" = 2
  dimension "d557" = 2
  dimension "d558" = 2
  dimension "d559" = 2
  dimension "d560" = 2
  dimension "d561" = 2
  dimension "d562" = 2
  dimension "d563" = 2
  dimension "d564" = 2
  dimension "d565" = 2
  dimension "d566" = 2
  dimension "d567" = 2
  dimension "d568" = 2
  dimension "d569" = 2
  dimension "d570" = 2
  dimension "d571" = 2
  dimension "d572" = 2
  dimension "d573" = 2
  dimension "d574" = 2
  dimension "d575" = 2
  dimension "d576" = 2
  dimension "d577" = 2
  dimension "d578" = 2
  dimension "d579" = 2
  dimension "d580" = 2
  dimension "d581" = 2
  dimension "d582" = 2
  dimension "d583" = 2
  dimension "d584" = 2
  dimension "d585" = 2
  dimension "d586" = 2
  dimension "d587" = 2
  dimension "d588" = 2
  dimension "d589" = 2
  dimension "d590" = 2
  dimension "d591" = 2
  dimension "d592" = 2
  dimension "d593" = 2
  dimension "d594" = 2
  dimension "d595" = 2
  dimension "d596" = 2
  dimension "d597" = 2
  dimension "d598" = 2
  dimension "d599" = 2
  dimension "d600" = 2
  dimension "d601" = 2
  dimension "d602" = 2
  dimension "d603" = 2
  dimension "d604" = 2
  dimension "d605" = 2
  dimension "d606" = 2
  dimension "d607" = 2
  dimension "d608" = 2
  dimension "d609" = 2
  dimension "d610" = 2
  dimension "d611" = 2
  dimension "d612" = 2
  dimension "d613" = 2
  dimension "d614" = 2
  dimension "d615" = 2
  dimension "d616" = 2
  dimension "d617" = 2
  dimension "d618" = 2
  dimension "d619" = 2
  dimension "d620" = 2
  dimension "d621" = 2
  dimension "d622" = 2
  dimension "d623" = 2
  dimension "d624" = 5
  measures "d131" diameter of A0
  measures "d132" diameter of A1
  measures "d138" diameter of A3
  measures "d139" diameter of A2
  measures "d142" diameter of A6
  measures "d143" diameter of A4
  measures "d144" diameter of A5
  measures "d145" diameter of A11
  measures "d146" diameter of A15
  measures "d147" diameter of A7
  measures "d148" diameter of A10
  measures "d149" diameter of A14
  measures "d150" diameter of A9
  measures "d151" diameter of A16
  measures "d152" diameter of A12
  measures "d153" diameter of A13
  measures "d154" diameter of A8
  measures "d155" diameter of A17
  measures "d159" diameter of A21
  measures "d160" diameter of A19
  measures "d166" diameter of A18
  measures "d167" diameter of A20
  measures "d170" diameter of A29
  measures "d171" diameter of A22
  measures "d172" diameter of A23
  measures "d173" diameter of A25
  measures "d174" diameter of A26
  measures "d175" diameter of A24
  measures "d176" diameter of A35
  measures "d177" diameter of A27
  measures "d178" diameter of A30
  measures "d179" diameter of A28
  measures "d180" diameter of A32
  measures "d181" diameter of A34
  measures "d182" diameter of A33
  measures "d183" diameter of A31
  measures "d185" diameter of A39
  measures "d187" diameter of A44
  measures "d188" diameter of A41
  measures "d189" diameter of A36
  measures "d190" diameter of A40
  measures "d191" diameter of A50
  measures "d192" diameter of A42
  measures "d194" diameter of A37
  measures "d195" diameter of A43
  measures "d196" diameter of A51
  measures "d197" diameter of A38
  measures "d198" diameter of A54
  measures "d199" diameter of A45
  measures "d200" diameter of A46
  measures "d201" diameter of A48
  measures "d202" diameter of A49
  measures "d203" diameter of A47
  measures "d204" diameter of A60
  measures "d205" diameter of A52
  measures "d206" diameter of A55
  measures "d207" diameter of A53
  measures "d208" diameter of A57
  measures "d209" diameter of A59
  measures "d210" diameter of A58
  measures "d211" diameter of A56
  measures "d212" diameter of A61
  measures "d213" diameter of A62
  measures "d215" diameter of A63
  measures "d216" diameter of A64
  measures "d217" diameter of A65
  measures "d218" diameter of A66
  measures "d219" diameter of A67
  measures "d220" diameter of A68
  measures "d221" diameter of A69
  measures "d222" diameter of A70
  measures "d223" diameter of A71
  measures "d224" diameter of A143
  measures "d225" diameter of A150
  measures "d226" diameter of A149 A45.centre
  measures "d227" diameter of A142
  measures "d228" diameter of A134
  measures "d231" diameter of A147
  measures "d233" diameter of A146
  measures "d234" diameter of A144
  measures "d235" diameter of A133
  measures "d238" diameter of A89
  measures "d239" diameter of A91
  measures "d240" diameter of A94
  measures "d241" diameter of A77
  measures "d242" diameter of A116
  measures "d243" diameter of A118
  measures "d244" diameter of A112
  measures "d245" diameter of A85
  measures "d246" diameter of A96
  measures "d247" diameter of A82
  measures "d248" diameter of A88
  measures "d249" diameter of A114
  measures "d250" diameter of A109
  measures "d251" diameter of A117
  measures "d252" diameter of A140
  measures "d253" diameter of A138
  measures "d254" diameter of A124
  measures "d255" diameter of A139
  measures "d256" diameter of A141
  measures "d261" diameter of A123
  measures "d262" diameter of A102
  measures "d263" diameter of A137
  measures "d265" diameter of A131
  measures "d266" diameter of A78
  measures "d267" diameter of A97
  measures "d268" diameter of A72
  measures "d269" diameter of A92
  measures "d270" diameter of A111
  measures "d271" diameter of A103
  measures "d272" diameter of A86
  measures "d273" diameter of A81
  measures "d274" diameter of A76
  measures "d275" diameter of A79
  measures "d276" diameter of A95
  measures "d277" diameter of A113
  measures "d278" diameter of A105
  measures "d279" diameter of A101
  measures "d283" diameter of A129
  measures "d284" diameter of A125
  measures "d285" diameter of A128
  measures "d286" diameter of A126
  measures "d290" diameter of A127
  measures "d291" diameter of A136
  measures "d292" diameter of A135
  measures "d293" diameter of A130
  measures "d294" diameter of A99
  measures "d295" diameter of A115
  measures "d296" diameter of A108
  measures "d297" diameter of A100
  measures "d298" diameter of A93
  measures "d299" diameter of A107
  measures "d300" diameter of A98
  measures "d301" diameter of A106
  measures "d302" diameter of A83
  measures "d303" diameter of A122
  measures "d304" diameter of A104
  measures "d305" diameter of A84
  measures "d306" diameter of A75
  measures "d307" diameter of A119
  measures "d308" diameter of A90
  measures "d309" diameter of A132
  measures "d311" diameter of A110
  measures "d312" diameter of A80
  measures "d313" diameter of A145
  measures "d314" diameter of A148
  measures "d315" diameter of A120
  measures "d316" diameter of A87
  measures "d317" diameter of A73
  measures "d318" diameter of A121
  measures "d319" diameter of A74
  measures "d320" distance of A40.centre A62.centre
  measures "d321" diameter of A175
  measures "d322" diameter of A163
  measures "d323" diameter of A221
  measures "d324" diameter of A165